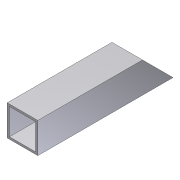
# Autodesk Inventor part: FE-00001-01
Saved by Autodesk Inventor 2012 (Build 160160000, 160)
## iProperties
Created: 2008-05-14
Part Number: FE-00001-01
Document SubType Name: Modeling
Designer: narosenberg
Density: 1 g/cm^3
Mass: 91.5371 g
Surface Area: 589.267 cm^2
Volume: 91.5371 cm^3
Description: Connector Tube
Material: Default
Author: narosenberg
Autodesk Inventor part; units mm, degrees
ref_plane "YZ Plane" through (0, 0, 0) normal (1, 0, 0) x (0, 1, 0)
ref_plane "XZ Plane" through (0, 0, 0) normal (0, 1, 0) x (-1, 0, 0)
ref_plane "XY Plane" through (0, 0, 0) normal (0, 0, 1) x (1, 0, 0)
sketch "Sketch1" plane through (0, 0, 0) normal (0, 0, 1) x (1, 0, 0)
  line L0 (-30.5992, 26.7179) -> (13.8508, 26.7179)
  line L1 (13.8508, 26.7179) -> (13.8508, -17.7321)
  line L2 (13.8508, -17.7321) -> (-30.5992, -17.7321)
  line L3 (-30.5992, -17.7321) -> (-30.5992, 26.7179)
  dimension "d0" = 44.45
  dimension "d1" = 44.45
  constraints: 8 end point, 2 parallel, 1 horizontal, 1 perpendicular
  measures "d0" distance of L0.end L1.end
  measures "d1" distance of L1.end L2.end
extrude "Extrusion1" add sketch "Sketch1" along normal blind 196.85
shell "Shell1" thickness 3.175 removed faces 2 at (-15.7825, -2.9154, 0) at (-15.7825, -2.9154, 196.85)
sketch "Sketch2" plane through (13.8508, -17.7321, 0) normal (1, 0, 0) x (0, 0, -1)
  line L0 (0, 0) -> (-196.85, 0) projected
  line L1 (0, 44.45) -> (0, 0) projected
  line L2 (0, 44.45) -> (-196.85, 44.45) projected
  line L3 (0, 0) -> (-44.45, 44.45)
  dimension "d5" = 45
  constraints: 2 end point, 1 point on line
  measures "d5" angle of L0 L3
extrude "Extrusion2" cut sketch "Sketch2" against normal through all
body "Solid1"
